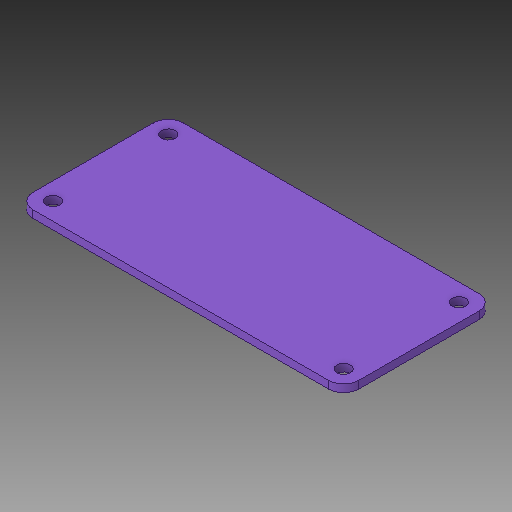
# Autodesk Inventor part: PiZeroWMechanicalLayout
Saved by Autodesk Inventor 2019.2 (Build 232265000, 265)
## iProperties
Created: 2018-12-18
Part Number: PiZeroWMechanicalLayout
Material: LCP Plastic
Document SubType Name: Modeling
Designer: steele
Density: 1.626 g/cm^3
Appearance: Violet
Author: steele
Autodesk Inventor part; units mm, degrees
ref_plane "YZ Plane" through (0, 0, 0) normal (1, 0, 0) x (0, 1, 0)
ref_plane "XZ Plane" through (0, 0, 0) normal (0, 1, 0) x (-1, 0, 0)
ref_plane "XY Plane" through (0, 0, 0) normal (0, 0, 1) x (1, 0, 0)
sketch "Sketch1" plane through (0, 0, 0) normal (0, 1, 0) x (-1, 0, 0)
  line L0 (32.5, 15) -> (-32.5, 15)
  line L1 (-32.5, 15) -> (-32.5, -15)
  line L2 (-32.5, -15) -> (32.5, -15)
  line L3 (32.5, -15) -> (32.5, 15)
  line L4 (32.5, 15) -> (-32.5, -15) construction
  line L5 (-32.5, 15) -> (32.5, -15) construction
  point P0 (0, 0)
  point P1 (-29, 11.5)
  point P2 (-29, -11.5)
  dimension "d0" = 65
  dimension "d1" = 30
  constraints: 12 end point, 2 midpoint, 2 parallel, 1 horizontal, 1 perpendicular
  measures "d0" distance of L0.start L0.end
  measures "d1" distance of L2.end L0.start
extrude "Extrusion1" add sketch "Sketch1" against normal blind 1.5
sketch "Sketch2" plane through (0, 0, 0) normal (0, 1, 0) x (1, 0, 0)
  line L0 (-29, -11.5) -> (29, -11.5) construction
  line L1 (29, -11.5) -> (29, 11.5) construction
  line L2 (29, 11.5) -> (-29, 11.5) construction
  line L3 (-29, 11.5) -> (-29, -11.5) construction
  line L4 (-29, -11.5) -> (29, 11.5) construction
  line L5 (29, -11.5) -> (-29, 11.5) construction
  point P0 (0, 0)
  dimension "d6" = 58
  dimension "d7" = 23
  constraints: 12 end point, 4 coincident, 2 midpoint, 2 parallel, 1 horizontal, 1 perpendicular
  measures "d6" distance of L0.start L0.end
  measures "d7" distance of L2.end L0.start
hole "Hole1" at (-29, 0, 11.5) at (-29, 0, -11.5) at (29, 0, -11.5) at (29, 0, 11.5) direction (0, -1, 0) diameter 2.75 end through all
fillet "Fillet1" radius 3 4 edges at (-32.5, -0.75, 15) (32.5, -0.75, 15) (32.5, -0.75, -15) (-32.5, -0.75, -15)
equation "\"d0\" = PiZeroWLength"
equation "\"d1\" = PiZeroWWidth"
equation "\"d4\" = PiZeroWHeight"
equation "\"d6\" = PiZeroMoutingHolesLength"
equation "\"d7\" = PiZeroMountingHolesWidth"
equation "\"d8\" = PiZeroWMountingHole"
equation "\"PiZeroWHeight\" = 1.5"
equation "\"PiZeroWLength\" = 65"
equation "\"PiZeroWWidth\" = 30"
equation "\"PiZeroMoutingHolesLength\" = 58"
equation "\"PiZeroMountingHolesWidth\" = 23"
equation "\"PiZeroWMountingHole\" = 2.75"
body "Solid1"
